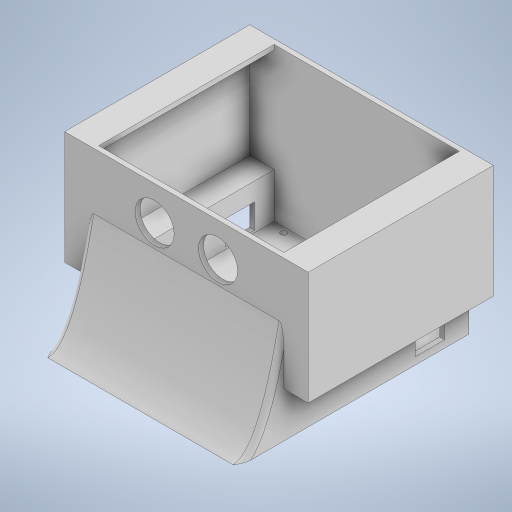
# Autodesk Inventor part: SUMOBOT
Saved by Autodesk Inventor 2024 (Build 280153000, 153)
## iProperties
Created: 2024-01-10
Part Number: SUMOBOT
Material: Generic
Document SubType Name: Modeling
Designer: Yuvraj
Density: 1 g/cm^3
Appearance: Default
Author: Yuvraj
Autodesk Inventor part; units mm, degrees
ref_plane "YZ Plane" through (0, 0, 0) normal (1, 0, 0) x (0, 1, 0)
ref_plane "XZ Plane" through (0, 0, 0) normal (0, 1, 0) x (-1, 0, 0)
ref_plane "XY Plane" through (0, 0, 0) normal (0, 0, 1) x (1, 0, 0)
sketch "Sketch2" plane through (0, 0, 0) normal (0, 1, 0) x (-1, 0, 0)
  point P0 (0, 0)
sketch "Sketch3" plane through (0, 0, 0) normal (0, 1, 0) x (-1, 0, 0)
  line L0 (40, 38) -> (-40, 38)
  line L1 (-40, 38) -> (-40, -38)
  line L2 (-40, -38) -> (40, -38)
  line L3 (40, -38) -> (40, 38)
  point P0 (0, 0)
  dimension "d0" = 38
  dimension "d1" = 38
  dimension "d2" = 40
  dimension "d3" = 40
  constraints: 8 end point, 2 parallel, 1 horizontal, 1 perpendicular
  measures "d0" distance from line of point (0, 0) L0
  measures "d1" distance from line of L2 point (0, 0)
  measures "d2" distance from line of point (0, 0) L3
  measures "d3" distance from line of point (0, 0) L1
extrude "Extrusion1" add sketch "Sketch3" along normal blind 65
shell "Shell1" thickness 2 removed faces 1 at (13.333333, 65, 12.666667)
sketch "Sketch8" plane through (40, 0, 38) normal (1, 0, 0) x (0, 0, -1)
  line L0 (66, 3) -> (53.95, 3)
  line L1 (53.95, 3) -> (53.95, 13.05)
  line L2 (53.95, 13.05) -> (66, 13.05)
  line L3 (66, 13.05) -> (66, 3)
  line L4 (0, 0) -> (76, 0) projected
  line L5 (76, 0) -> (76, 65) projected
  point P0 (38, 0)
  dimension "d18" = 10.05
  dimension "d19" = 12.05
  dimension "d20" = 13.05
  dimension "d44" = 10
  constraints: 8 end point, 2 parallel, 1 horizontal, 1 perpendicular
  measures "d18" distance of L0.end L1.end
  measures "d19" distance of L0.start L0.end
  measures "d20" distance between parallel lines of L4 L2
  measures "d44" distance between parallel lines of L5 L3
extrude "Extrusion4" cut sketch "Sketch8" against normal blind 90
sketch "Sketch10" plane through (-40, 0, -38) normal (-1, 0, 0) x (0, 0, 1)
  line L0 (0, 0) -> (0, 65) projected
  line L1 (76, 0) -> (76, 65) projected
  line L2 (0, 65) -> (76, 65)
  line L3 (76, 65) -> (76, 18.5)
  line L4 (76, 18.5) -> (0, 18.5)
  line L5 (0, 18.5) -> (0, 65)
  point P0 (38, 0)
  point P1 (0, 18.5)
  dimension "d28" = 46.5
  constraints: 8 end point, 2 parallel, 1 horizontal, 1 perpendicular, 1 point on line
  measures "d28" distance between parallel lines of L2 L4
extrude "Extrusion5" add sketch "Sketch10" along normal blind 10
sketch "Sketch11" plane through (40, 0, 38) normal (1, 0, 0) x (0, 0, -1)
  line L0 (0, 65) -> (76, 65) projected
  line L1 (76, 65) -> (76, 18.5) projected
  line L2 (0, 65) -> (76, 65)
  line L3 (76, 65) -> (76, 18.5)
  line L4 (76, 18.5) -> (0, 18.5)
  line L5 (0, 18.5) -> (0, 65)
  point P0 (38, 0)
  constraints: 8 end point, 2 parallel, 1 horizontal, 1 perpendicular
extrude "Extrusion6" add sketch "Sketch11" along normal blind 10
shell "Shell2" thickness 2 removed faces 2 at (38, 47.683333, -5.316667) at (-38, 47.683333, -5.316667)
sketch "Sketch12" plane through (0, 0, 0) normal (1, 0, 0) x (0, 1, 0)
  line L0 (18.5, 38) -> (65, 38)
  spline S0 degree 2 poles (41.75, 38) (-0.109895, 46.486594) (0, 57) knots 0 0 0 1 1 1
  line L1 (0, 57) -> (0, 38)
  line L2 (0, 38) -> (41.75, 38)
  line L3 (20.5, 36) -> (63, 36)
  line L4 (65, 38) -> (18.5, 38)
  point P0 (0, 0)
  point P1 (3.554834, 51)
  point P2 (41.75, 38)
  point P3 (0, 56.889941)
  dimension "d34" = 6
  dimension "d35" = 13
  constraints: 4 end point, 2 midpoint, 1 parallel, 1 vertical, 3 other
  measures "d34" vertical distance of point (3.555, 51) L1.start
  measures "d35" vertical distance of point (41.75, 38) point (3.555, 51)
sketch "Sketch12 outline for Extrusion7" plane through (0, 0, 0) normal (1, 0, 0) x (0, 1, 0)
  line L0 (0, 38) -> (18.5, 38)
  line L1 (0, 56.889941) -> (0, 38)
  spline S0 degree 2 poles (41.75, 38) (0.109319, 46.442151) (0, 56.889941) knots 0 0 0 1 1 1
  line L2 (18.5, 38) -> (41.75, 38)
extrude "Extrusion7" add sketch "Sketch12 outline for Extrusion7" along normal mid plane 80
fillet "Fillet2" radius 2 2 edges at (40, 10.4922, 46.9436) (-40, 10.4922, 46.9436)
sketch "Sketch13" plane through (-50, 18.5, 38) normal (0, 0, 1) x (1, 0, 0)
  circle A0 centre (36.95, 32.5) radius 8.025
  circle A1 centre (63, 32.5) radius 8.025
  line L0 (100, 46.5) -> (0, 46.5) projected
  line L1 (100, 46.5) -> (100, 0) projected
  line L2 (44.975, 32.5) -> (54.975, 32.5)
  point P0 (50, -18.5)
  dimension "d39" = 16.05
  dimension "d40" = 16.05
  dimension "d41" = 26.05
  dimension "d72" = 14
  dimension "d73" = 14
  dimension "d74" = 37
  dimension "d75" = 10
  constraints: 2 end point, 2 horizontal alignment, 4 other
  measures "d41" distance of point (63, 32.5) point (36.95, 32.5)
  measures "d72" distance from line of L0 point (36.95, 32.5)
  measures "d73" distance from line of L0 point (63, 32.5)
  measures "d74" distance from line of L1 point (63, 32.5)
  measures "d75" distance of L2.start L2.end
extrude "Extrusion8" cut sketch "Sketch13" against normal blind 2
sketch "Sketch15" plane through (0, 0, 0) normal (0, -1, 0) x (1, 0, 0)
  circle A0 centre (-32, -16) radius 1.25
  circle A1 centre (-32, -34) radius 1.25
  circle A2 centre (32, -16) radius 1.25
  circle A3 centre (32, -34) radius 1.25
  line L0 (-40, -38) -> (-40, 51.71657)
  line L1 (40, 51.71657) -> (40, -38)
  line L2 (40, -38) -> (-40, -38)
  point P0 (0, 0)
  dimension "d45" = 18
  dimension "d46" = 18
  dimension "d47" = 8
  dimension "d49" = 8
  dimension "d50" = 8
  dimension "d51" = 8
  dimension "d52" = 4
  dimension "d53" = 4
  dimension "d54" = 2.5
  dimension "d55" = 2.5
  dimension "d56" = 2.5
  dimension "d57" = 2.5
  constraints: 4 centre point
  measures "d45" distance of A1.centre A0.centre
  measures "d46" distance of A3.centre A2.centre
  measures "d47" distance from line of L0 A1.centre
  measures "d49" distance from line of L0 A0.centre
  measures "d50" distance from line of L1 A2.centre
  measures "d51" distance from line of L1 A3.centre
  measures "d52" distance from line of L2 A1.centre
  measures "d53" distance from line of L2 A3.centre
  measures "d54" diameter of A3
  measures "d55" diameter of A2
  measures "d56" diameter of A0
  measures "d57" diameter of A1
extrude "Extrusion9" cut sketch "Sketch15" against normal blind 10
sketch "Sketch16" plane through (40, 18.5, -38) normal (0, -1, 0) x (1, 0, 0)
  line L0 (8, 74) -> (8, 2)
  line L1 (2, 72) -> (8, 72)
  line L2 (8, 72) -> (8, 60)
  line L3 (8, 60) -> (2, 60)
  line L4 (2, 60) -> (2, 72)
  line L5 (0, 89.71657) -> (0, 0)
  line L6 (0, 76) -> (10, 76)
  point P0 (-40, 38)
  point P1 (8, 72)
  dimension "d60" = 2
  dimension "d61" = 4
  dimension "d62" = 16
  constraints: 8 end point, 2 parallel, 1 horizontal, 1 perpendicular, 1 point on line
  measures "d60" distance between parallel lines of L5 L4
  measures "d61" distance between parallel lines of L6 L1
  measures "d62" distance between parallel lines of L6 L3
sketch "Sketch17" plane through (-40, 18.5, -38) normal (0, -1, 0) x (1, 0, 0)
  line L0 (-2, 72) -> (-8, 72)
  line L1 (-8, 72) -> (-8, 60)
  line L2 (-8, 60) -> (-2, 60)
  line L3 (-2, 60) -> (-2, 72)
  line L4 (0, 76) -> (-10, 76) projected
  line L5 (-10, 0) -> (-10, 76) projected
  point P0 (40, 38)
  point P1 (-2, 66)
  dimension "d63" = 4
  dimension "d64" = 16
  dimension "d65" = 2
  dimension "d66" = 8
  constraints: 8 end point, 2 parallel, 1 horizontal, 1 midpoint, 1 perpendicular
  measures "d63" distance between parallel lines of L4 L0
  measures "d64" distance between parallel lines of L4 L2
  measures "d65" distance between parallel lines of L5 L1
  measures "d66" distance from line of L5 point (-2, 66)
extrude "Extrusion10" cut sketch "Sketch17" against normal blind 10
extrude "Extrusion11" cut sketch "Sketch16" against normal blind 10
body "Solid1"
